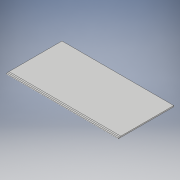
# Autodesk Inventor part: Arbeitsplatte
Saved by Autodesk Inventor 2017 (Build 210142000, 142)
## iProperties
Created: 2017-06-01
Part Number: Arbeitsplatte
Material: Generic
Document SubType Name: Modeling
Designer: Fake
Density: 1 g/cm^3
Appearance: Default
Author: Fake
Autodesk Inventor part; units mm, degrees
ref_plane "YZ Plane" through (0, 0, 0) normal (1, 0, 0) x (0, 1, 0)
ref_plane "XZ Plane" through (0, 0, 0) normal (0, 1, 0) x (-1, 0, 0)
ref_plane "XY Plane" through (0, 0, 0) normal (0, 0, 1) x (1, 0, 0)
sketch "Skizze1" plane through (0, 0, 0) normal (1, 0, 0) x (0, 1, 0)
  line L0 (-291.0081, 0) -> (1108.9919, 0) projected
  line L1 (0, -4) -> (0, 24) projected
  line L2 (-91.0081, 20) -> (908.9919, 20)
  line L3 (908.9919, 20) -> (908.9919, 0)
  line L4 (908.9919, 0) -> (-91.0081, 0)
  line L5 (-91.0081, 0) -> (-91.0081, 20)
  line L6 (-51.0081, 20) -> (-91.0081, 10)
  dimension "d0" = 20
  dimension "d1" = 1000
  dimension "d2" = 40
  dimension "d3" = 10
  constraints: 10 end point, 2 parallel, 1 collinear, 1 horizontal, 1 midpoint, 1 perpendicular, 1 point on line
  measures "d0" distance between parallel lines of L2 L4
  measures "d1" distance of L2.start L2.end
  measures "d2" distance from line of L5 L6.start
  measures "d3" distance from line of L2 L6.end
extrude "Extrusion1" add sketch "Skizze1" along normal mid plane 2000 contours L5 L6 L2 L1 L0 | L1 L2 L3 L0
fillet "Rundung1" radius 100 1 edges at (0, -51.0081, 20)
fillet "Rundung2" radius 6 2 edges at (0, -91.0081, 10) (0, -91.0081, 0)
